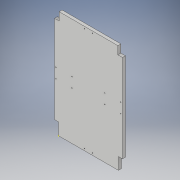
# Autodesk Inventor part: Arm Belly Pan
Saved by Autodesk Inventor 2018 (Build 220112000, 112)
## iProperties
Created: 2019-01-30
Part Number: Arm Belly Pan
Material: Generic
Document SubType Name: Modeling
Designer: maste
Density: 1 g/cm^3
Appearance: Default
Author: maste
Autodesk Inventor part; units mm, degrees
ref_plane "YZ Plane" through (0, 0, 0) normal (1, 0, 0) x (0, 1, 0)
ref_plane "XZ Plane" through (0, 0, 0) normal (0, 1, 0) x (-1, 0, 0)
ref_plane "XY Plane" through (0, 0, 0) normal (0, 0, 1) x (1, 0, 0)
sketch "Sketch1" plane through (0, 0, 0) normal (0, 0, 1) x (1, 0, 0)
  line L0 (0, 0) -> (0, 76.2)
  line L1 (0, 76.2) -> (-25.4, 76.2)
  line L2 (-25.4, 76.2) -> (-25.4, 635)
  line L3 (-25.4, 635) -> (3.175, 635)
  line L4 (3.175, 635) -> (3.175, 685.8)
  line L5 (3.175, 685.8) -> (377.825, 685.8)
  line L6 (377.825, 685.8) -> (377.825, 635)
  line L7 (377.825, 635) -> (406.4, 635)
  line L8 (406.4, 635) -> (406.4, 76.2)
  line L9 (406.4, 76.2) -> (381, 76.2)
  line L10 (381, 76.2) -> (381, 0)
  line L11 (381, 0) -> (0, 0)
  dimension "d0" = 76.2
  dimension "d1" = 25.4
  dimension "d2" = 558.8
  dimension "d3" = 28.575
  dimension "d4" = 50.8
  dimension "d5" = 374.65
  dimension "d6" = 28.575
  dimension "d7" = 25.4
  constraints: 24 end point, 9 perpendicular, 2 point on line, 2 vertical
  measures "d0" distance of L0.start L0.end
  measures "d1" distance of L0.end L1.end
  measures "d2" distance of L1.end L2.end
  measures "d3" distance of L2.end L3.end
  measures "d4" distance of L3.end L4.end
  measures "d5" distance of L4.end L5.end
  measures "d6" distance of L6.end L7.end
  measures "d7" distance of L8.end L9.end
extrude "Extrusion1" add sketch "Sketch1" along normal blind 19.05
sketch "Sketch2" plane through (0, 0, 19.05) normal (0, 0, 1) x (1, 0, 0)
  point P0 (0, 0)
sketch "Sketch3" plane through (0, 0, 19.05) normal (0, 0, 1) x (1, 0, 0)
  line L0 (-25.4, 635) -> (-25.4, 76.2) construction
  line L1 (-25.4, 635) -> (-25.4, 369.062) construction
  line L2 (-25.4, 369.062) -> (-16.9333, 369.062) construction
  line L3 (-25.4, 369.062) -> (-16.9333, 369.062) construction
  line L4 (-16.9333, 369.062) -> (84.6667, 369.062) construction
  line L5 (-25.4, 76.2) -> (-25.4, 306.324) construction
  line L6 (-25.4, 306.324) -> (-16.9333, 306.324) construction
  line L7 (-16.9333, 306.324) -> (84.6667, 306.324) construction
  circle A0 centre (84.6667, 369.062) radius 2.5797
  circle A1 centre (-16.9333, 369.062) radius 2.5797
  circle A2 centre (84.6667, 306.324) radius 2.5797
  circle A3 centre (-16.9333, 306.324) radius 2.5797
  line L8 (377.825, 685.8) -> (3.175, 685.8) construction
  line L9 (190.5, 685.8) -> (190.5, 0) construction
  line L10 (0, 0) -> (381, 0) construction
  line L11 (190.5, 0) -> (165.1, 0) construction
  line L12 (165.1, 0) -> (165.1, 12.7) construction
  circle A4 centre (165.1, 12.7) radius 2.5797
  line L13 (190.5, 685.8) -> (165.1, 685.8) construction
  line L14 (165.1, 685.8) -> (165.1, 673.1) construction
  circle A5 centre (165.1, 673.1) radius 2.5797
  line L15 (406.4, 635) -> (406.4, 76.2) construction
  line L16 (406.4, 635) -> (406.4, 369.062) construction
  line L17 (406.4, 76.2) -> (406.4, 306.324) construction
  line L18 (3.175, 685.8) -> (377.825, 685.8) construction
  line L19 (381, 0) -> (0, 0) construction
  line L20 (190.5, 0) -> (215.9, 0) construction
  line L21 (215.9, 0) -> (215.9, 12.7) construction
  circle A6 centre (215.9, 12.7) radius 2.5797
  line L22 (190.5, 685.8) -> (215.9, 685.8) construction
  line L23 (215.9, 685.8) -> (215.9, 673.1) construction
  circle A7 centre (215.9, 673.1) radius 2.5797
  line L24 (406.4, 76.2) -> (406.4, 635) projected
  line L25 (406.4, 685.8) -> (406.4, 382.5189) construction
  line L26 (406.4, 382.5189) -> (395.1148, 382.5189) construction
  line L27 (395.1148, 382.5189) -> (293.5148, 382.5189) construction
  line L28 (293.5148, 382.5189) -> (293.5148, 319.7809) construction
  line L29 (293.5148, 319.7809) -> (395.1148, 319.7809) construction
  circle A8 centre (395.1148, 382.5189) radius 2.5797
  circle A9 centre (293.5148, 382.5189) radius 2.5797
  circle A10 centre (293.5148, 319.7809) radius 2.5797
  circle A11 centre (395.1148, 319.7809) radius 2.5797
  dimension "d10" = 265.938
  dimension "d11" = 8.4667
  dimension "d12" = 0
  dimension "d13" = 101.6
  dimension "d14" = 230.124
  dimension "d15" = 5.1594
  dimension "d16" = 25.4
  dimension "d17" = 12.7
  dimension "d19" = 5.1594
  dimension "d20" = 25.4
  dimension "d21" = 12.7
  dimension "d25" = 303.2811
  dimension "d26" = 11.2852
  dimension "d27" = 101.6
  dimension "d28" = 62.738
  dimension "d29" = 5.1594
  constraints: 52 end point, 14 symmetric about line, 12 centre point, 12 coincident, 11 point on line, 4 horizontal, 4 perpendicular, 2 midpoint, 1 collinear, 1 vertical, 2 other
  measures "d10" distance of L0.start L1.end
  measures "d11" distance of L1.end L2.end
  measures "d12" distance between parallel lines of L2 L3
  measures "d13" distance of L2.end L4.end
  measures "d14" distance of L0.end L5.end
  measures "d15" diameter of A0
  measures "d16" distance of L9.end L11.end
  measures "d17" distance of L11.end L12.end
  measures "d19" diameter of A4
  measures "d20" distance of L9.start L13.end
  measures "d21" distance of L13.end L14.end
  measures "d25" distance of L25.start L25.end
  measures "d26" distance of L25.end L26.end
  measures "d27" distance of L26.end L27.end
  measures "d28" distance of L27.end L28.end
  measures "d29" diameter of A8
extrude "Extrusion2" cut sketch "Sketch3" against normal blind 25.4
body "Solid1"
